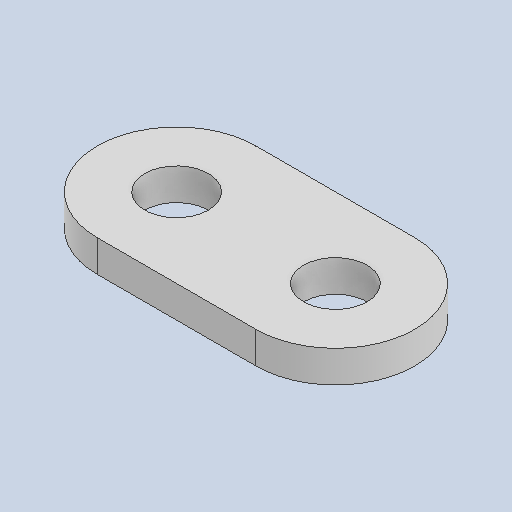
# Autodesk Inventor part: T Slot Nut
Saved by Autodesk Inventor 2023 (Build 270158000, 158)
## iProperties
Created: 2022-10-04
Part Number: T Slot Nut
Material: Generic
Document SubType Name: Modeling
Designer: Raker
Density: 1 g/cm^3
Appearance: Default
Author: Raker
Autodesk Inventor part; units mm, degrees
ref_plane "YZ Plane" through (0, 0, 0) normal (1, 0, 0) x (0, 1, 0)
ref_plane "XZ Plane" through (0, 0, 0) normal (0, 1, 0) x (-1, 0, 0)
ref_plane "XY Plane" through (0, 0, 0) normal (0, 0, 1) x (1, 0, 0)
sketch "Sketch1" plane through (0, 0, 0) normal (0, 1, 0) x (-1, 0, 0)
  arc A0 (5, -5) -> (5, 5) centre (5, 0) ccw
  arc A1 (-5, 5) -> (-5, -5) centre (-5, 0) ccw
  line L0 (0, -7) -> (0, 7) projected
  line L1 (5, -5) -> (-5, -5)
  line L2 (5, 5) -> (-5, 5)
  circle A2 centre (5, 0) radius 2
  circle A3 centre (-5, 0) radius 2
  point P0 (0, 0)
  point P1 (-10, 0)
  point P2 (10, 0)
  dimension "d0" = 10
  dimension "d1" = 4
  dimension "d3" = 20
  constraints: 6 point on circle, 4 centre point, 4 end point, 2 coincident, 2 equal radius, 2 tangent, 1 horizontal alignment, 1 parallel, 1 other
  measures "d0" diameter of A0
  measures "d1" diameter of A3
  measures "d3" distance of point (-10, 0) point (10, 0)
extrude "Extrusion1" add sketch "Sketch1" along normal blind 2
body "Solid1"
